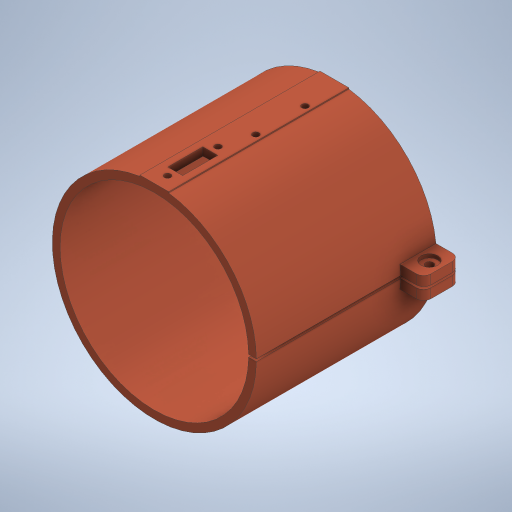
# Autodesk Inventor part: sensor_adapter
Saved by Autodesk Inventor 2023 (Build 270158000, 158)
## iProperties
Created: 2023-10-19
Part Number: sensor_adapter
Material: Generic
Document SubType Name: Modeling
Designer: mark
Density: 1 g/cm^3
Appearance: Default
Author: mark
Autodesk Inventor part; units mm, degrees
ref_plane "YZ Plane" through (0, 0, 0) normal (1, 0, 0) x (0, 1, 0)
ref_plane "XZ Plane" through (0, 0, 0) normal (0, 1, 0) x (-1, 0, 0)
ref_plane "XY Plane" through (0, 0, 0) normal (0, 0, 1) x (1, 0, 0)
sketch "Sketch1" plane through (0, 0, 0) normal (0, 0, 1) x (1, 0, 0)
  circle A0 centre (0, 0) radius 39.25
  circle A1 centre (0, 0) radius 42.5
  line L0 (39.2468, 0.5) -> (42.4971, 0.5)
  line L1 (44.2943, 0.5) -> (44.2943, -0.5)
  line L2 (42.497, -0.5013) -> (39.2468, -0.5013)
  line L3 (38.2943, -0.5) -> (38.2943, 0.5)
  line L4 (-6, 42.55) -> (6, 42.55)
  line L5 (6, 42.55) -> (6, 38.73)
  line L6 (6, 38.73) -> (-6, 38.73)
  line L7 (-6, 38.73) -> (-6, 42.55)
  point P0 (-6, 42.0743)
  point P1 (6, 42.0743)
  dimension "d0" = 78.5
  dimension "d1" = 85
  dimension "d2" = 6
  dimension "d3" = 1
  dimension "d4" = 0.5
  dimension "d7" = 12
  dimension "d8" = 6
  dimension "d9" = 42.55
  constraints: 16 end point, 4 parallel, 4 point on circle, 2 centre point, 2 coincident, 2 horizontal, 2 perpendicular
  measures "d0" diameter of A0
  measures "d1" diameter of A1
  measures "d2" distance of L1.end L3.start
  measures "d3" distance of L1.start L1.end
  measures "d4" distance from line of point (0, 0) L0
  measures "d7" distance of L4.start L4.end
  measures "d8" distance from line of point (0, 0) L5
  measures "d9" distance from line of point (0, 0) L4
extrude "Extrusion1" add sketch "Sketch1" along normal blind 75 contours A0 L5 A1 L0 | L2 A1 L7 A0 | A0 L7 A1 L5 | A1 L7 L4 L5
sketch "Sketch3" plane through (39.2468, 0.5, 0) normal (0, -1, 0) x (1, 0, 0)
  line L0 (3.2502, 0) -> (-33.2468, 0) projected
  line L1 (2.9121, 0) -> (9.9121, 0)
  line L2 (12.9121, 3) -> (12.9121, 12)
  line L3 (9.9121, 15) -> (2.9121, 15)
  line L4 (2.9121, 15) -> (2.9121, 0)
  arc A0 (12.9121, 12) -> (9.9121, 15) centre (9.9121, 12) ccw
  arc A1 (9.9121, 0) -> (12.9121, 3) centre (9.9121, 3) ccw
  point P0 (-39.2468, 0)
  point P1 (12.9121, 15)
  point P2 (12.9121, 0)
  dimension "d10" = 10
  dimension "d11" = 15
  dimension "d12" = 3
  constraints: 8 end point, 5 point on line, 4 point on circle, 4 tangent, 2 centre point, 2 parallel, 1 equal radius, 1 horizontal, 1 perpendicular
  measures "d10" distance of L3.end point (12.912, 15)
  measures "d11" distance of point (12.912, 15) point (12.912, 0)
  measures "d12" radius of A0
extrude "Extrusion2" add sketch "Sketch3" against normal blind 4
sketch "Sketch4" plane through (39.2468, 4.5, 0) normal (0, 1, 0) x (1, 0, 0)
  circle A0 centre (7.8143, -7.5) radius 3.5
  line L0 (9.9121, 0) -> (3.0143, 0) projected
  line L1 (3.0143, -15) -> (3.0143, 0) projected
  point P0 (-39.2468, 0)
  point P1 (3.0143, -7.5)
  dimension "d15" = 7
  dimension "d16" = 7.5
  dimension "d17" = 4.8
  constraints: 1 centre point, 1 midpoint
  measures "d15" diameter of A0
  measures "d16" distance from line of L0 A0.centre
  measures "d17" distance of point (3.014, -7.5) A0.centre
extrude "Extrusion3" cut sketch "Sketch4" against normal blind 1.5
sketch "Sketch5" plane through (47.0611, 3, 7.5) normal (0, 1, 0) x (1, 0, 0)
  circle A0 centre (0, 0) radius 3.5 projected
  point P0 (-47.0611, 7.5)
  constraints: 1 coincident
hole "Hole1" at (47.0611, 3, 7.5) direction (0, -1, 0) diameter 3.2 end through all
mirror "Mirror1" about plane through (0, 0, 0) normal (0, 1, 0) of "Extrusion2", "Extrusion3", "Hole1"
sketch "Sketch6" plane through (-6, 42.55, 0) normal (0, 1, 0) x (1, 0, 0)
  line L0 (0, 0) -> (0, -75) projected
  line L1 (12, 0) -> (12, -75) projected
  line L2 (0, -13) -> (12, -13)
  line L3 (12, -13) -> (12, -39)
  line L4 (12, -39) -> (0, -39)
  line L5 (0, -39) -> (0, -13)
  circle A0 centre (9.5, -15.75) radius 1.35
  circle A1 centre (9.5, -36.25) radius 1.35
  line L6 (12, 0) -> (0, 0) projected
  line L7 (2.9, -72) -> (9.1, -72)
  line L8 (9.1, -72) -> (9.1, -46)
  line L9 (9.1, -46) -> (2.9, -46)
  line L10 (2.9, -46) -> (2.9, -72)
  line L11 (12, -75) -> (0, -75) projected
  circle A2 centre (6, -69.5) radius 1.35
  circle A3 centre (6, -48.5) radius 1.35
  line L12 (2.9, -51.7) -> (9.1, -51.7)
  line L13 (9.1, -51.7) -> (9.1, -66.3)
  line L14 (9.1, -66.3) -> (2.9, -66.3)
  line L15 (2.9, -66.3) -> (2.9, -51.7)
  point P0 (6, 0)
  point P1 (6, -46)
  point P2 (2.9, -66.3)
  point P3 (9.1, -51.7)
  dimension "d27" = 26
  dimension "d28" = 2.7
  dimension "d29" = 2.7
  dimension "d30" = 2.75
  dimension "d31" = 2.5
  dimension "d32" = 2.5
  dimension "d33" = 2.75
  dimension "d34" = 13
  dimension "d35" = 6.2
  dimension "d36" = 26
  dimension "d37" = 2.9
  dimension "d38" = 3
  dimension "d39" = 2.7
  dimension "d40" = 2.7
  dimension "d41" = 2.5
  dimension "d42" = 2.5
  dimension "d43" = 3.1
  dimension "d44" = 3.1
  dimension "d47" = 14.6
  dimension "d48" = 5.7
  constraints: 24 end point, 6 parallel, 4 centre point, 4 point on line, 3 horizontal, 3 perpendicular, 1 midpoint
  measures "d27" distance of L2.end L3.end
  measures "d28" diameter of A0
  measures "d29" diameter of A1
  measures "d30" distance from line of L2 A0.centre
  measures "d31" distance from line of L1 A0.centre
  measures "d32" distance from line of L1 A1.centre
  measures "d33" distance from line of L4 A1.centre
  measures "d34" distance between parallel lines of L6 L2
  measures "d35" distance of L9.end L8.end
  measures "d36" distance of L8.end L7.end
  measures "d37" distance between parallel lines of L0 L10
  measures "d38" distance between parallel lines of L11 L7
  measures "d39" diameter of A2
  measures "d40" diameter of A3
  measures "d41" distance of point (6, -46) A3.centre
  measures "d42" distance from line of L7 A2.centre
  measures "d43" distance from line of L8 A2.centre
  measures "d44" distance from line of L8 A3.centre
  measures "d47" distance of L12.end L13.end
  measures "d48" distance between parallel lines of L9 L12
extrude "Extrusion4" cut sketch "Sketch6" against normal blind 6 contours A0 | A1 | L10 L12 L8 L14 | A2 | A3
chamfer "Chamfer1" distance 1 angle 45 1 edges at (-39.25, 0.0006, 0)
equation "\"d8\" = 0.5 * d7"
equation "\"d29\" = d28"
equation "\"d32\" = d31"
equation "\"d33\" = d30"
equation "\"d40\" = d39"
equation "\"d41\" = d42"
equation "\"d44\" = d43"
body "Solid1"
